Autodesk Inventor part; units mm, degrees
(part 2 of 2)
  spline S284 degree 2 poles (-0.0848, -12.3603) (0.1178, -12.3603) (0.4735, -12.3998) (0.6068, -12.4443) knots 0 0 0 1 2 2 2
  line L262 (0.6068, -12.4443) -> (0.6068, -13.2297)
  line L263 (0.6068, -13.2297) -> (0.5723, -13.2297)
  spline S285 degree 2 poles (0.5723, -13.2297) (0.4586, -13.1705) (0.0437, -13.0667) (-0.1934, -13.0667) knots 0 0 0 1 2 2 2
  spline S286 degree 2 poles (-0.1934, -13.0667) (-0.9542, -13.0667) (-1.8879, -14.0942) (-1.9768, -15.102) knots 0 0 0 1 2 2 2
  spline S287 degree 2 poles (-1.9768, -15.102) (-1.6853, -14.8995) (-1.0728, -14.6772) (-0.7072, -14.6772) knots 0 0 0 1 2 2 2
  spline S288 degree 2 poles (-0.7072, -14.6772) (-0.3515, -14.6772) (0.182, -14.8204) (0.4735, -15.0378) knots 0 0 0 1 2 2 2
  spline S289 degree 2 poles (0.4735, -15.0378) (0.8094, -15.2897) (1.1354, -16.0703) (1.1354, -16.5939) knots 0 0 0 1 2 2 2
  spline S290 degree 2 poles (0.3055, -16.6285) (0.3055, -16.253) (0.1079, -15.7442) (-0.1095, -15.5664) knots 0 0 0 1 2 2 2
  spline S291 degree 2 poles (-0.1095, -15.5664) (-0.2725, -15.4379) (-0.6776, -15.3539) (-0.89, -15.3539) knots 0 0 0 1 2 2 2
  spline S292 degree 2 poles (-0.89, -15.3539) (-1.1765, -15.3539) (-1.715, -15.5268) (-1.9768, -15.6899) knots 0 0 0 1 2 2 2
  spline S293 degree 2 poles (-1.9768, -15.6899) (-1.9817, -15.7788) (-1.9916, -15.9468) (-1.9916, -16.0752) knots 0 0 0 1 2 2 2
  spline S294 degree 2 poles (-1.9916, -16.0752) (-1.9916, -16.7075) (-1.7446, -17.4831) (-1.5569, -17.6856) knots 0 0 0 1 2 2 2
  spline S295 degree 2 poles (-1.5569, -17.6856) (-1.384, -17.8783) (-1.0085, -18.0314) (-0.7961, -18.0314) knots 0 0 0 1 2 2 2
  spline S296 degree 2 poles (-0.7961, -18.0314) (-0.3021, -18.0314) (0.3055, -17.33) (0.3055, -16.6285) knots 0 0 0 1 2 2 2
  line L264 (4.3909, -12.2022) -> (2.0049, -19.8938)
  line L265 (2.0049, -19.8938) -> (1.3133, -19.8938)
  line L266 (1.3133, -19.8938) -> (3.6894, -12.2022)
  line L267 (3.6894, -12.2022) -> (4.3909, -12.2022)
  line L268 (8.8221, -18.5699) -> (5.0628, -18.5699)
  line L269 (5.0628, -18.5699) -> (5.0628, -17.7054)
  spline S297 degree 2 poles (5.0628, -17.7054) (5.4678, -17.325) (6.1891, -16.6186) (6.5349, -16.2382) knots 0 0 0 1 2 2 2
  spline S298 degree 2 poles (6.5349, -16.2382) (7.2314, -15.4725) (7.7403, -14.5537) (7.7403, -14.0646) knots 0 0 0 1 2 2 2
  spline S299 degree 2 poles (7.7403, -14.0646) (7.7403, -13.8077) (7.5822, -13.4224) (7.4389, -13.2989) knots 0 0 0 1 2 2 2
  spline S300 degree 2 poles (7.4389, -13.2989) (7.2957, -13.1754) (6.9202, -13.0519) (6.693, -13.0519) knots 0 0 0 1 2 2 2
  spline S301 degree 2 poles (6.693, -13.0519) (6.4756, -13.0519) (6.031, -13.1606) (5.8285, -13.2446) knots 0 0 0 1 2 2 2
  spline S302 degree 2 poles (5.8285, -13.2446) (5.6556, -13.3137) (5.3345, -13.5113) (5.2357, -13.5805) knots 0 0 0 1 2 2 2
  line L270 (5.2357, -13.5805) -> (5.1912, -13.5805)
  line L271 (5.1912, -13.5805) -> (5.1912, -12.711)
  spline S303 degree 2 poles (5.1912, -12.711) (5.4431, -12.5875) (6.3472, -12.3455) (6.7522, -12.3455) knots 0 0 0 1 2 2 2
  spline S304 degree 2 poles (6.7522, -12.3455) (7.6069, -12.3455) (8.5702, -13.2495) (8.5702, -14.0201) knots 0 0 0 1 2 2 2
  spline S305 degree 2 poles (8.5702, -14.0201) (8.5702, -14.3808) (8.4022, -14.9834) (8.254, -15.2403) knots 0 0 0 1 2 2 2
  spline S306 degree 2 poles (8.254, -15.2403) (8.1058, -15.5071) (7.676, -16.0307) (7.4389, -16.2827) knots 0 0 0 1 2 2 2
  spline S307 degree 2 poles (7.4389, -16.2827) (7.0536, -16.7026) (6.11, -17.6017) (5.8285, -17.8635) knots 0 0 0 1 2 2 2
  line L272 (5.8285, -17.8635) -> (8.8221, -17.8635)
  line L273 (8.8221, -17.8635) -> (8.8221, -18.5699)
  spline S308 degree 2 poles (13.4312, -15.5219) (13.4312, -17.162) (12.4777, -18.6984) (11.4848, -18.6984) knots 0 0 0 1 2 2 2
  spline S309 degree 2 poles (11.4848, -18.6984) (10.477, -18.6984) (9.5335, -17.1324) (9.5335, -15.5268) knots 0 0 0 1 2 2 2
  spline S310 degree 2 poles (9.5335, -15.5268) (9.5335, -13.8769) (10.4869, -12.3504) (11.4848, -12.3504) knots 0 0 0 1 2 2 2
  spline S311 degree 2 poles (11.4848, -12.3504) (12.4876, -12.3504) (13.4312, -13.9312) (13.4312, -15.5219) knots 0 0 0 1 2 2 2
  spline S312 degree 2 poles (12.3839, -17.3794) (12.5024, -17.078) (12.6012, -16.1493) (12.6012, -15.5219) knots 0 0 0 1 2 2 2
  spline S313 degree 2 poles (12.6012, -15.5219) (12.6012, -14.8945) (12.5024, -13.9707) (12.3789, -13.6595) knots 0 0 0 1 2 2 2
  spline S314 degree 2 poles (12.3789, -13.6595) (12.2554, -13.3483) (11.8257, -13.0272) (11.4848, -13.0272) knots 0 0 0 1 2 2 2
  spline S315 degree 2 poles (11.4848, -13.0272) (11.1439, -13.0272) (10.7043, -13.3483) (10.5758, -13.6694) knots 0 0 0 1 2 2 2
  spline S316 degree 2 poles (10.5758, -13.6694) (10.4523, -13.9806) (10.3634, -14.9291) (10.3634, -15.5268) knots 0 0 0 1 2 2 2
  spline S317 degree 2 poles (10.3634, -15.5268) (10.3634, -16.1691) (10.4425, -17.0286) (10.5709, -17.3645) knots 0 0 0 1 2 2 2
  spline S318 degree 2 poles (10.5709, -17.3645) (10.6895, -17.6807) (11.1291, -18.0216) (11.4848, -18.0216) knots 0 0 0 1 2 2 2
  spline S319 degree 2 poles (11.4848, -18.0216) (11.8207, -18.0216) (12.2604, -17.7005) (12.3839, -17.3794) knots 0 0 0 1 2 2 2
  line L274 (17.9711, -18.5699) -> (14.2117, -18.5699)
  line L275 (14.2117, -18.5699) -> (14.2117, -17.7054)
  spline S320 degree 2 poles (14.2117, -17.7054) (14.6168, -17.325) (15.338, -16.6186) (15.6838, -16.2382) knots 0 0 0 1 2 2 2
  spline S321 degree 2 poles (15.6838, -16.2382) (16.3804, -15.4725) (16.8892, -14.5537) (16.8892, -14.0646) knots 0 0 0 1 2 2 2
  spline S322 degree 2 poles (16.8892, -14.0646) (16.8892, -13.8077) (16.7311, -13.4224) (16.5879, -13.2989) knots 0 0 0 1 2 2 2
  spline S323 degree 2 poles (16.5879, -13.2989) (16.4446, -13.1754) (16.0692, -13.0519) (15.8419, -13.0519) knots 0 0 0 1 2 2 2
  spline S324 degree 2 poles (15.8419, -13.0519) (15.6245, -13.0519) (15.1799, -13.1606) (14.9774, -13.2446) knots 0 0 0 1 2 2 2
  spline S325 degree 2 poles (14.9774, -13.2446) (14.8045, -13.3137) (14.4834, -13.5113) (14.3846, -13.5805) knots 0 0 0 1 2 2 2
  line L276 (14.3846, -13.5805) -> (14.3401, -13.5805)
  line L277 (14.3401, -13.5805) -> (14.3401, -12.711)
  spline S326 degree 2 poles (14.3401, -12.711) (14.5921, -12.5875) (15.4961, -12.3455) (15.9012, -12.3455) knots 0 0 0 1 2 2 2
  spline S327 degree 2 poles (15.9012, -12.3455) (16.7558, -12.3455) (17.7191, -13.2495) (17.7191, -14.0201) knots 0 0 0 1 2 2 2
  spline S328 degree 2 poles (17.7191, -14.0201) (17.7191, -14.3808) (17.5512, -14.9834) (17.403, -15.2403) knots 0 0 0 1 2 2 2
  spline S329 degree 2 poles (17.403, -15.2403) (17.2548, -15.5071) (16.825, -16.0307) (16.5879, -16.2827) knots 0 0 0 1 2 2 2
  spline S330 degree 2 poles (16.5879, -16.2827) (16.2025, -16.7026) (15.259, -17.6017) (14.9774, -17.8635) knots 0 0 0 1 2 2 2
  line L278 (14.9774, -17.8635) -> (17.9711, -17.8635)
  line L279 (17.9711, -17.8635) -> (17.9711, -18.5699)
  spline S331 degree 2 poles (22.4813, -16.6334) (22.4813, -17.0731) (22.1997, -17.824) (21.9428, -18.1006) knots 0 0 0 1 2 2 2
  spline S332 degree 2 poles (21.9428, -18.1006) (21.686, -18.3772) (20.9203, -18.6984) (20.446, -18.6984) knots 0 0 0 1 2 2 2
  spline S333 degree 2 poles (20.446, -18.6984) (20.0113, -18.6984) (19.1616, -18.5057) (18.8504, -18.3525) knots 0 0 0 1 2 2 2
  line L280 (18.8504, -18.3525) -> (18.8504, -17.488)
  line L281 (18.8504, -17.488) -> (18.9097, -17.488)
  spline S334 degree 2 poles (18.9097, -17.488) (19.0035, -17.5572) (19.3543, -17.735) (19.5667, -17.8141) knots 0 0 0 1 2 2 2
  spline S335 degree 2 poles (19.5667, -17.8141) (19.8088, -17.8981) (20.2089, -17.9919) (20.4608, -17.9919) knots 0 0 0 1 2 2 2
  spline S336 degree 2 poles (20.4608, -17.9919) (20.7078, -17.9919) (21.1722, -17.8141) (21.3402, -17.6214) knots 0 0 0 1 2 2 2
  spline S337 degree 2 poles (21.3402, -17.6214) (21.4933, -17.4386) (21.6514, -16.9545) (21.6514, -16.6285) knots 0 0 0 1 2 2 2
  spline S338 degree 2 poles (21.6514, -16.6285) (21.6514, -16.3024) (21.4735, -15.8875) (21.3056, -15.7492) knots 0 0 0 1 2 2 2
  spline S339 degree 2 poles (21.3056, -15.7492) (21.1327, -15.596) (20.6189, -15.4676) (20.3077, -15.4676) knots 0 0 0 1 2 2 2
  spline S340 degree 2 poles (20.3077, -15.4676) (19.9718, -15.4676) (19.3049, -15.5713) (19.1023, -15.6158) knots 0 0 0 1 2 2 2
  line L282 (19.1023, -15.6158) -> (19.1023, -12.4739)
  line L283 (19.1023, -12.4739) -> (22.4467, -12.4739)
  line L284 (22.4467, -12.4739) -> (22.4467, -13.1902)
  line L285 (22.4467, -13.1902) -> (19.8878, -13.1902)
  line L286 (19.8878, -13.1902) -> (19.8878, -14.8155)
  spline S341 degree 2 poles (19.8878, -14.8155) (20.036, -14.7957) (20.3225, -14.7809) (20.4411, -14.7809) knots 0 0 0 1 2 2 2
  spline S342 degree 2 poles (20.4411, -14.7809) (20.9104, -14.7809) (21.5575, -14.934) (21.8539, -15.1613) knots 0 0 0 1 2 2 2
  spline S343 degree 2 poles (21.8539, -15.1613) (22.1553, -15.3885) (22.4813, -16.0801) (22.4813, -16.6334) knots 0 0 0 1 2 2 2
  line L287 (3.5931, -28.6068) -> (2.6841, -28.6068)
  line L288 (2.6841, -28.6068) -> (-0.0131, -23.3506)
  line L289 (-0.0131, -23.3506) -> (-0.0131, -28.6068)
  line L290 (-0.0131, -28.6068) -> (-0.769, -28.6068)
  line L291 (-0.769, -28.6068) -> (-0.769, -22.5108)
  line L292 (-0.769, -22.5108) -> (0.3821, -22.5108)
  line L293 (0.3821, -22.5108) -> (2.8373, -27.3372)
  line L294 (2.8373, -27.3372) -> (2.8373, -22.5108)
  line L295 (2.8373, -22.5108) -> (3.5931, -22.5108)
  line L296 (3.5931, -22.5108) -> (3.5931, -28.6068)
  point P0 (0, 0)
  constraints: 2 other
emboss "Emboss1" sketch "Sketch2" operation cut depth 2.54 direction (-1, 0, 0)
sketch "Sketch3" plane through (0, 0, 0) normal (-1, 0, 0) x (0, 0, 1)
  line L0 (-2.1568, 3.0969) -> (3.484, 3.0969) construction
  line L1 (3.484, 3.0969) -> (3.484, -5.309) construction
  line L2 (3.484, -5.309) -> (-2.1568, -5.309) construction
  line L3 (-2.1568, -5.309) -> (-2.1568, 3.0969) construction
  spline S0 degree 2 poles (0.1601, -3.2164) (-0.5019, -3.2164) (-1.4306, -2.9398) (-1.8406, -2.7422) knots 0 0 0 1 2 2 2
  line L4 (-1.8406, -2.7422) -> (-1.8406, -1.7246)
  line L5 (-1.8406, -1.7246) -> (-1.7813, -1.7246)
  spline S1 degree 2 poles (-1.7813, -1.7246) (-1.3812, -2.1) (-0.3685, -2.515) (0.1008, -2.515) knots 0 0 0 1 2 2 2
  spline S2 degree 2 poles (0.1008, -2.515) (0.7727, -2.515) (1.4593, -1.9567) (1.4593, -1.4973) knots 0 0 0 1 2 2 2
  spline S3 degree 2 poles (1.4593, -1.4973) (1.4593, -1.1318) (1.0987, -0.6773) (0.7084, -0.5637) knots 0 0 0 1 2 2 2
  spline S4 degree 2 poles (0.7084, -0.5637) (0.4269, -0.4846) (-0.0424, -0.3759) (-0.3932, -0.287) knots 0 0 0 1 2 2 2
  spline S5 degree 2 poles (-0.3932, -0.287) (-0.7093, -0.203) (-1.2083, 0.0489) (-1.401, 0.2515) knots 0 0 0 1 2 2 2
  spline S6 degree 2 poles (-1.401, 0.2515) (-1.5887, 0.454) (-1.7962, 0.9974) (-1.7962, 1.3531) knots 0 0 0 1 2 2 2
  spline S7 degree 2 poles (-1.7962, 1.3531) (-1.7962, 2.0941) (-0.6402, 3.0969) (0.254, 3.0969) knots 0 0 0 1 2 2 2
  spline S8 degree 2 poles (0.254, 3.0969) (0.7677, 3.0969) (1.6767, 2.8944) (2.0669, 2.7017) knots 0 0 0 1 2 2 2
  line L6 (2.0669, 2.7017) -> (2.0669, 1.7335)
  line L7 (2.0669, 1.7335) -> (2.0077, 1.7335)
  spline S9 degree 2 poles (2.0077, 1.7335) (1.7162, 2.0002) (0.8072, 2.3954) (0.3083, 2.3954) knots 0 0 0 1 2 2 2
  spline S10 degree 2 poles (0.3083, 2.3954) (-0.2549, 2.3954) (-0.9514, 1.8668) (-0.9514, 1.4371) knots 0 0 0 1 2 2 2
  spline S11 degree 2 poles (-0.9514, 1.4371) (-0.9514, 1.0517) (-0.5414, 0.5923) (-0.1561, 0.4886) knots 0 0 0 1 2 2 2
  spline S12 degree 2 poles (-0.1561, 0.4886) (0.1008, 0.4194) (0.8468, 0.2416) (1.0938, 0.1675) knots 0 0 0 1 2 2 2
  spline S13 degree 2 poles (1.0938, 0.1675) (1.7211, -0.0252) (2.3041, -0.8008) (2.3041, -1.3689) knots 0 0 0 1 2 2 2
  spline S14 degree 2 poles (2.3041, -1.3689) (2.3041, -1.7295) (2.0126, -2.4211) (1.7508, -2.6632) knots 0 0 0 1 2 2 2
  spline S15 degree 2 poles (1.7508, -2.6632) (1.4593, -2.9299) (0.7183, -3.2164) (0.1601, -3.2164) knots 0 0 0 1 2 2 2
  point P0 (0, 0)
  constraints: 2 other
emboss "Emboss2" sketch "Sketch3" operation cut depth 2.54 direction (1, 0, 0)
body "Solid1"
